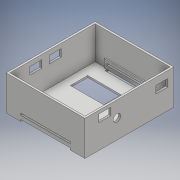
# Autodesk Inventor part: chest_piece_bottom_2
Saved by Autodesk Inventor 2017 (Build 210142000, 142)
## iProperties
Created: 2017-05-08
Part Number: chest_piece_bottom_2
Material: Generic
Document SubType Name: Modeling
Designer: Gabe Madonna
Density: 1 g/cm^3
Appearance: Default
Author: Gabe Madonna
Autodesk Inventor part; units mm, degrees
ref_plane "YZ Plane" through (0, 0, 0) normal (1, 0, 0) x (0, 1, 0)
ref_plane "XZ Plane" through (0, 0, 0) normal (0, 1, 0) x (-1, 0, 0)
ref_plane "XY Plane" through (0, 0, 0) normal (0, 0, 1) x (1, 0, 0)
sketch "Sketch1" plane through (0, 0, 0) normal (0, 0, 1) x (1, 0, 0)
  line L0 (-41, -46.5) -> (41, -46.5)
  line L1 (41, -46.5) -> (41, 46.5)
  line L2 (41, 46.5) -> (-41, 46.5)
  line L3 (-41, 46.5) -> (-41, -46.5)
  line L4 (-41, -46.5) -> (41, 46.5) construction
  line L5 (41, -46.5) -> (-41, 46.5) construction
  line L6 (43, 48.5) -> (43, -48.5)
  line L7 (43, -48.5) -> (-43, -48.5)
  line L8 (-43, -48.5) -> (-43, 48.5)
  line L9 (-43, 48.5) -> (43, 48.5)
  point P0 (0, 0)
  dimension "d0" = 93
  dimension "d1" = 82
  dimension "d2" = 2
  constraints: 20 end point, 4 parallel, 2 midpoint, 2 perpendicular, 1 horizontal, 3 other
  measures "d0" distance of L0.end L1.end
  measures "d1" distance of L1.end L2.end
  measures "d2" distance between parallel lines of L1 L6
extrude "Extrusion1" add sketch "Sketch1" along normal blind 40
sketch "Sketch2" plane through (0, 0, 0) normal (0, 0, -1) x (-1, 0, 0)
  line L0 (41, 46.5) -> (41, -46.5) projected
  line L1 (41, -46.5) -> (-41, -46.5) projected
  line L2 (-41, -46.5) -> (-41, 46.5) projected
  line L3 (-41, 46.5) -> (41, 46.5) projected
  line L4 (-43, 48.5) -> (-43, -48.5) projected
  line L5 (-43, -48.5) -> (43, -48.5) projected
  line L6 (43, -48.5) -> (43, 48.5) projected
  line L7 (43, 48.5) -> (-43, 48.5) projected
  point P0 (0, 0)
extrude "Extrusion2" add sketch "Sketch2" along normal blind 2 contours L0 L1 L2 L3 | L7 L6 L5 L4
sketch "Sketch4" plane through (0, 0, -2) normal (0, 0, -1) x (-1, 0, 0)
  line L0 (41, 46.5) -> (41, -46.5) projected
  line L1 (-41, 46.5) -> (41, 46.5) projected
  line L2 (-41, -46.5) -> (-41, 46.5) projected
  line L3 (41, -46.5) -> (-41, -46.5) projected
  line L4 (0, 46.5) -> (0, 31.5)
  line L5 (41, -46.5) -> (41, 46.5) projected
  line L6 (41, 31.5) -> (37, 31.5)
  line L7 (-41, 46.5) -> (-41, -46.5) projected
  line L8 (-41, 16) -> (-7, 16)
  line L9 (23, -46.5) -> (23, 3.5)
  line L10 (37, 31.5) -> (-10, 31.5)
  line L11 (-10, 31.5) -> (-10, 3.5)
  line L12 (-10, 3.5) -> (37, 3.5)
  line L13 (37, 3.5) -> (37, 31.5)
  point P0 (0, 0)
  dimension "d11" = 15
  dimension "d12" = 4
  dimension "d13" = 34
  dimension "d14" = 50
  constraints: 16 end point, 3 perpendicular, 3 point on line, 2 parallel, 2 vertical, 1 horizontal, 1 midpoint
  measures "d11" distance of L4.start L4.end
  measures "d12" distance of L6.start L6.end
  measures "d13" distance of L8.start L8.end
  measures "d14" distance of L9.start L9.end
extrude "Extrusion4" cut sketch "Sketch4" against normal blind 2 contours L13 L12 L11 L10
sketch "Sketch8" plane through (-43, 48.5, 40) normal (0, 1, 0) x (1, 0, 0)
  line L0 (0, 0) -> (0, 42) projected
  line L1 (86, 0) -> (0, 0) projected
  line L2 (86, 42) -> (86, 0) projected
  line L3 (0, 42) -> (86, 42) projected
  line L4 (6, 42) -> (53, 42) projected
  line L5 (43, 42) -> (16, 42)
  line L6 (43, 42) -> (43, 40)
  line L7 (43, 40) -> (43, 36)
  line L8 (43, 36) -> (43, 34)
  line L9 (84, 40) -> (2, 40) projected
  line L10 (16, 42) -> (70, 42)
  line L11 (70, 42) -> (70, 40)
  line L12 (70, 40) -> (16, 40)
  line L13 (16, 40) -> (16, 42)
  line L14 (16, 34) -> (70, 34)
  line L15 (70, 34) -> (70, 36)
  line L16 (70, 36) -> (16, 36)
  line L17 (16, 36) -> (16, 34)
  dimension "d29" = 27
  dimension "d30" = 2
  dimension "d31" = 4
  dimension "d32" = 2
  dimension "d33" = 54
  constraints: 24 end point, 5 point on line, 4 parallel, 3 perpendicular, 2 horizontal
  measures "d29" distance of L5.start L5.end
  measures "d30" distance of L5.start L6.end
  measures "d31" distance of L6.end L7.end
  measures "d32" distance of L7.end L8.end
  measures "d33" distance of L11.end L12.end
sketch "Sketch9" plane through (-43, 48.5, 40) normal (0, 1, 0) x (1, 0, 0)
  line L0 (70, 42) -> (73, 42)
  line L1 (6, 42) -> (53, 42) projected
  line L2 (16, 42) -> (13, 42)
  line L3 (70, 34) -> (70, 31)
  line L4 (73, 42) -> (13, 42)
  line L5 (13, 42) -> (13, 31)
  line L6 (13, 31) -> (73, 31)
  line L7 (73, 31) -> (73, 42)
  point P0 (43, 40)
  dimension "d34" = 3
  dimension "d35" = 3
  dimension "d36" = 3
  constraints: 14 end point, 2 horizontal, 2 parallel, 2 point on line, 1 perpendicular, 1 vertical
  measures "d34" distance of L0.start L0.end
  measures "d35" distance of L2.start L2.end
  measures "d36" distance of L3.start L3.end
extrude "Extrusion8" add sketch "Sketch9" against normal blind 3
extrude "Extrusion9" cut sketch "Sketch8" against normal blind 5 contours L16 L15 L14 L8 | L8 L14 L17 L16 | L3 L6 L9 L13 | L11 L9 L6 L3
sketch "Sketch10" plane through (0, 0, 40) normal (0, 0, 1) x (1, 0, 0)
  line L0 (-41, -46.5) -> (-41, 46.5) projected
  line L1 (-41, 46.5) -> (41, 46.5) projected
  line L2 (41, 46.5) -> (41, -46.5) projected
  line L3 (41, -46.5) -> (-41, -46.5) projected
  line L4 (43, -48.5) -> (43, 48.5) projected
  line L5 (43, 48.5) -> (-43, 48.5) projected
  line L6 (-43, 48.5) -> (-43, -48.5) projected
  line L7 (-43, -48.5) -> (43, -48.5) projected
  point P0 (0, 0)
extrude "Extrusion10" cut sketch "Sketch10" against normal blind 4
sketch "Sketch11" plane through (-43, -48.5, -2) normal (-1, 0, 0) x (0, 0, 1)
  line L0 (2, 95) -> (38, 95) projected
  line L1 (2, 95) -> (2, 2) projected
  line L2 (11, 95) -> (2, 95) projected
  line L3 (2, 95) -> (2, 62.2)
  line L4 (2, 80) -> (2, 52) projected
  line L5 (2, 62.2) -> (21, 62.2)
  circle A0 centre (21, 62.2) radius 4
  line L6 (2, 79) -> (30.5, 79)
  line L7 (30.5, 95) -> (30.5, 83)
  line L8 (30.5, 83) -> (30.5, 72)
  line L9 (30.5, 79) -> (30.5, 72)
  line L10 (26.5, 82) -> (34.5, 82)
  line L11 (34.5, 82) -> (34.5, 69)
  line L12 (34.5, 69) -> (26.5, 69)
  line L13 (26.5, 69) -> (26.5, 82)
  line L14 (26.5, 82) -> (34.5, 69) construction
  line L15 (34.5, 82) -> (26.5, 69) construction
  line L16 (2, 7) -> (26.5, 7)
  line L17 (2, 2) -> (38, 2) projected
  line L18 (26.42, 2) -> (26.42, 13.2)
  line L19 (22.42, 6.7) -> (22.42, 19.7)
  line L20 (22.42, 19.7) -> (30.42, 19.7)
  line L21 (30.42, 19.7) -> (30.42, 6.7)
  line L22 (30.42, 6.7) -> (22.42, 6.7)
  line L23 (22.42, 6.7) -> (30.42, 19.7) construction
  line L24 (22.42, 19.7) -> (30.42, 6.7) construction
  line L25 (2, 2) -> (38, 2) projected
  line L26 (2, 95) -> (2, 2)
  line L27 (2, 2) -> (2, 48.5)
  line L28 (2, 2) -> (2, 95) projected
  line L29 (28, 48.5) -> (2, 48.5)
  circle A1 centre (21, 34.8) radius 4
  line L30 (26.5, 15) -> (34.5, 15)
  line L31 (34.5, 15) -> (34.5, 28)
  line L32 (34.5, 28) -> (26.5, 28)
  line L33 (26.5, 28) -> (26.5, 15)
  line L34 (22.42, 90.3) -> (22.42, 77.3)
  line L35 (22.42, 77.3) -> (30.42, 77.3)
  line L36 (30.42, 77.3) -> (30.42, 90.3)
  line L37 (30.42, 90.3) -> (22.42, 90.3)
  point P0 (30.5, 75.5)
  dimension "d43" = 32.8
  dimension "d44" = 19
  dimension "d45" = 8
  dimension "d48" = 28.5
  dimension "d50" = 12
  dimension "d51" = 11
  dimension "d52" = 8
  dimension "d53" = 13
  dimension "d54" = 24.5
  dimension "d55" = 11.2
  dimension "d56" = 13
  dimension "d57" = 8
  constraints: 62 end point, 9 symmetric about line, 6 perpendicular, 6 point on line, 5 midpoint, 5 vertical, 4 parallel, 2 centre point, 1 coincident, 1 collinear, 1 horizontal, 1 other
  measures "d43" distance of L0.start L3.end
  measures "d44" distance of L3.end L5.end
  measures "d45" diameter of A0
  measures "d48" distance of L6.start L6.end
  measures "d50" distance of L7.start L7.end
  measures "d51" distance of L7.end L8.end
  measures "d52" distance of L10.start L10.end
  measures "d53" distance of L10.end L11.end
  measures "d54" distance of L16.start L16.end
  measures "d55" distance of L18.start L18.end
  measures "d56" distance of L19.start L19.end
  measures "d57" distance of L19.end L20.end
extrude "Extrusion11" cut sketch "Sketch11" against normal through all contours L34 L37 L36 L10 L13 L6 | L6 L13 L35 L34 | L13 L10 L36 L6 | L6 L36 L35 L13 | L33 L32 L31 L30 L21 L20 | L20 L21 L30 L33 | A1
sketch "Sketch12" plane through (-43, -48.5, -2) normal (-1, 0, 0) x (0, 0, 1)
  line L0 (38, 0) -> (38, 97) projected
  line L1 (38, 97) -> (0, 97) projected
  line L2 (0, 0) -> (0, 97) projected
  line L3 (38, 0) -> (0, 0) projected
  point P0 (2, 48.5)
extrude "Extrusion12" add sketch "Sketch12" against normal up to surface (2 mm away)
sketch "Sketch13" plane through (-43, -48.5, -2) normal (-1, 0, 0) x (0, 0, 1)
  line L0 (38, 0) -> (38, 97) projected
  line L1 (38, 97) -> (0, 97) projected
  line L2 (38, 0) -> (0, 0) projected
  line L3 (2, 95) -> (38, 95) projected
  line L4 (2, 95) -> (2, 2) projected
  line L5 (2, 2) -> (38, 2) projected
  line L6 (2, 72) -> (29, 72)
  line L7 (29.0235, 95) -> (29.0235, 51.4)
  line L8 (25.0235, 57.9) -> (33.0235, 57.9)
  line L9 (33.0235, 57.9) -> (33.0235, 44.9)
  line L10 (33.0235, 44.9) -> (25.0235, 44.9)
  line L11 (25.0235, 44.9) -> (25.0235, 57.9)
  line L12 (25.0235, 57.9) -> (33.0235, 44.9) construction
  line L13 (33.0235, 57.9) -> (25.0235, 44.9) construction
  line L14 (29.0235, 51.4) -> (29.0235, 30.4)
  line L15 (25.0235, 36.9) -> (33.0235, 36.9)
  line L16 (33.0235, 36.9) -> (33.0235, 23.9)
  line L17 (33.0235, 23.9) -> (25.0235, 23.9)
  line L18 (25.0235, 23.9) -> (25.0235, 36.9)
  line L19 (25.0235, 36.9) -> (33.0235, 23.9) construction
  line L20 (33.0235, 36.9) -> (25.0235, 23.9) construction
  line L21 (0, 0) -> (0, 97) projected
  point P0 (2, 48.5)
  dimension "d60" = 27
  dimension "d61" = 43.6
  dimension "d62" = 8
  dimension "d63" = 13
  dimension "d64" = 21
  dimension "d65" = 8
  dimension "d66" = 13
  constraints: 30 end point, 4 midpoint, 4 parallel, 3 horizontal, 2 perpendicular, 2 point on line, 2 vertical
  measures "d60" distance of L6.start L6.end
  measures "d61" distance of L7.start L7.end
  measures "d62" distance of L8.start L8.end
  measures "d63" distance of L8.end L9.end
  measures "d64" distance of L7.end L14.end
  measures "d65" distance of L15.start L15.end
  measures "d66" distance of L15.end L16.end
extrude "Extrusion13" cut sketch "Sketch13" against normal blind 8 contours L15 L16 L17 L18 | L8 L9 L10 L14 L7 | L7 L14 L10 L11 L8
mirror "Mirror3" about plane through (0, 0, 0) normal (0, 1, 0) of "Extrusion8", "Extrusion9"
sketch "Sketch14" plane through (0, 0, -2) normal (0, 0, -1) x (-1, 0, 0)
  line L0 (-27, -48.5) -> (-27, -43.5) projected
  line L1 (-27, -43.5) -> (27, -43.5) projected
  line L2 (27, -43.5) -> (27, -48.5) projected
  line L3 (27, -48.5) -> (43, -48.5) projected
  line L4 (43, -48.5) -> (43, 48.5) projected
  line L5 (43, 48.5) -> (27, 48.5) projected
  line L6 (27, 48.5) -> (27, 43.5) projected
  line L7 (27, 43.5) -> (-27, 43.5) projected
  line L8 (-27, 43.5) -> (-27, 48.5) projected
  line L9 (-27, 48.5) -> (-43, 48.5) projected
  line L10 (-43, 48.5) -> (-43, -48.5) projected
  line L11 (-43, -48.5) -> (-27, -48.5) projected
  line L12 (-41, -46.5) -> (-41, 46.5) projected
  line L13 (-41, 46.5) -> (-30, 46.5) projected
  line L14 (30, 46.5) -> (41, 46.5) projected
  line L15 (-30, 46.5) -> (-30, 45.5) projected
  line L16 (-4.5, 29.5) -> (32, 29.5)
  line L17 (32, 29.5) -> (32, 10.5)
  line L18 (32, 10.5) -> (-4.5, 10.5)
  line L19 (-4.5, 10.5) -> (-4.5, 29.5)
  line L20 (-10, 3.5) -> (-10, 31.5) projected
  line L21 (-10, 31.5) -> (37, 31.5) projected
  line L22 (37, 31.5) -> (37, 3.5) projected
  line L23 (37, 3.5) -> (-10, 3.5) projected
  constraints: 8 end point, 2 parallel, 1 horizontal, 1 perpendicular
extrude "Extrusion14" add sketch "Sketch14" against normal up to surface (2 mm away) contours L20 L21 L22 L23
body "Solid1"
